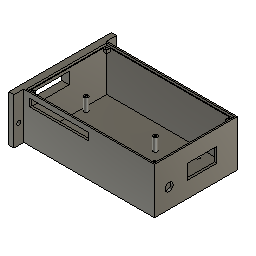
ComputeControlModule v6 (Autodesk Fusion 360 design; units mm, degrees)
Autodesk Fusion 360 part; units mm, degrees
sketch "Sketch1" plane through (0, 0, 0) normal (0, 0, 1) x (1, 0, 0)
  line L0 (0, 0) -> (178, 0)
  line L1 (178, 0) -> (178, 113)
  line L2 (178, 113) -> (0, 113)
  line L3 (0, 113) -> (0, 0)
  dimension "d1" = 178
  dimension "d2" = 113
  constraint horizontal L0
  constraint vertical L1
  constraint horizontal L2
  constraint vertical L3
  constraint coincident L0.start L3.end
  measures "d1" distance of L0.start L0.end
  measures "d2" distance of L0.start L2.end
extrude "Extrude1" add sketch "Sketch1" along normal blind 3
extrude "Extrude2" add 1 faces at (59.3333, 37.6667, 3) along direction (0, 0, 1) blind 60 thin wall 3 inside
sketch "Sketch2" plane through (0, 0, 0) normal (-1, 0, 0) x (0, -1, 0)
  line L0 (-113, 0) -> (0, 0)
  line L1 (0, 0) -> (0, 63)
  line L2 (0, 63) -> (-113, 63)
  line L3 (-113, 63) -> (-113, 0)
  line L4 (13.35, 0) -> (-126.35, 0)
  line L5 (-126.35, 0) -> (-126.35, 63)
  line L6 (-126.35, 63) -> (13.35, 63)
  line L7 (13.35, 63) -> (13.35, 0)
  line L8 (13.35, 0) -> (-126.35, 63) construction
  line L9 (-126.35, 0) -> (13.35, 63) construction
  point P0 (-56.5, 31.5)
  dimension "d8" = 139.7
  dimension "d9" = 63
  constraint horizontal L4
  constraint perpendicular L4 L5
  constraint parallel L4 L6
  constraint parallel L5 L7
  constraint coincident L8 P0
  constraint coincident L9 P0
  measures "d8" distance of L5.end L6.end
  measures "d9" distance of L4.end L5.end
extrude "Extrude3" add sketch "Sketch2" along normal blind 7
sketch "Sketch3" plane through (-7, 0, 0) normal (-1, 0, 0) x (0, -1, 0)
  line L0 (13.35, 63) -> (-126.35, 63)
  line L1 (-126.35, 63) -> (-126.35, 0)
  line L2 (-126.35, 0) -> (13.35, 0)
  line L3 (13.35, 0) -> (13.35, 63)
  point P0 (-120, 26.5)
  point P1 (7, 26.5)
hole "Hole1" at (-7, 120, 26.5) at (-7, -7, 26.5) direction (1, 0, 0) diameter 5.5 depth 12 tip angle 118
sketch "Sketch15" plane through (0, 0, 3) normal (0, 0, 1) x (-1, 0, 0)
  line L0 (-175, -110) -> (-3, -110)
  line L1 (-3, -110) -> (-3, -3)
  line L2 (-3, -3) -> (-175, -3)
  line L3 (-175, -3) -> (-175, -110)
  circle A0 centre (-102, -8) radius 3
  circle A1 centre (-102, -77) radius 3
  circle A2 centre (-8, -8) radius 3
  circle A3 centre (-8, -77) radius 3
  point P0 (-8, -8)
  point P1 (-8, -77)
  point P2 (-102, -8)
  point P3 (-102, -77)
  dimension "d103" = 6
  dimension "d104" = 6
  dimension "d105" = 6
  dimension "d106" = 6
  constraint coincident P2 A0.centre
  constraint coincident P3 A1.centre
  constraint coincident P0 A2.centre
  constraint coincident P1 A3.centre
  measures "d103" diameter of A0
  measures "d104" diameter of A1
  measures "d105" diameter of A2
  measures "d106" diameter of A3
extrude "Extrude13" add sketch "Sketch15" along normal blind 17 contours A0 | A1 | A2 | A3
sketch "Sketch16" plane through (0, 0, 20) normal (0, 0, 1) x (-1, 0, 0)
  circle A0 centre (-102, -8) radius 3
  point P0 (-102, -8)
  point P1 (-8, -8)
  point P2 (-8, -77)
  point P3 (-102, -77)
  constraint coincident P0 A0.centre
hole "Hole14" at (102, 77, 20) at (102, 8, 20) at (8, 8, 20) at (8, 77, 20) direction (0, 0, -1) diameter 2.75 depth 10 tip angle 180
sketch "Sketch17" plane through (0, 0, 3) normal (0, 0, 1) x (-1, 0, 0)
  circle A0 centre (-102, -77) radius 3
  circle A1 centre (-102, -8) radius 3
  circle A2 centre (-8, -77) radius 3
  circle A3 centre (-8, -8) radius 3
  line L0 (-175, -110) -> (-3, -110)
  line L1 (-3, -110) -> (-3, -3)
  line L2 (-3, -3) -> (-175, -3)
  line L3 (-175, -3) -> (-175, -110)
  circle A4 centre (-139, -8) radius 3
  circle A5 centre (-139, -98) radius 3
  point P0 (-139, -8)
  point P1 (-139, -98)
  dimension "d112" = 6
  dimension "d113" = 6
  constraint vertical P0 P1
  constraint coincident P0 A4.centre
  constraint coincident P1 A5.centre
  measures "d112" diameter of A4
  measures "d113" diameter of A5
extrude "Extrude14" add sketch "Sketch17" along normal blind 3 contours A4 | A5
sketch "Sketch18" plane through (0, 0, 6) normal (0, 0, 1) x (-1, 0, 0)
  circle A0 centre (-139, -8) radius 3
  point P0 (-139, -8)
  point P1 (-139, -98)
  constraint coincident P0 A0.centre
  constraint vertical P0 P1
hole "Hole15" at (139, 8, 6) at (139, 98, 6) direction (0, 0, -1) diameter 2.75 depth 4 tip angle 180
sketch "Sketch12" plane through (0, 0, 63) normal (0, 0, 1) x (-1, 0, 0)
  line L0 (-3, -110) -> (-175, -110)
  line L1 (-175, -110) -> (-175, -3)
  line L2 (-175, -3) -> (-3, -3)
  line L3 (-3, -3) -> (-3, -110)
  line L4 (0, 0) -> (-178, 0)
  line L5 (-178, 0) -> (-178, -113)
  line L6 (-178, -113) -> (0, -113)
  line L7 (-2, -111) -> (-176, -111)
  line L8 (-176, -111) -> (-176, -2)
  line L9 (-176, -2) -> (-2, -2)
  line L10 (-2, -2) -> (-2, -111)
  line L11 (0, -113) -> (0, -126.35)
  line L12 (0, -126.35) -> (7, -126.35)
  line L13 (7, -126.35) -> (7, 13.35)
  line L14 (7, 13.35) -> (0, 13.35)
  line L15 (0, 13.35) -> (0, 0)
  constraint horizontal L7
  constraint vertical L8
  constraint horizontal L9
  constraint vertical L10
extrude "Extrude11" cut sketch "Sketch12" against normal blind 3 contours L7 L8 L9 L10
ref_plane "WorkPlane1" through (85.5, 56.5, 61) normal (0, 0, 1) x (1, 0, 0)
sketch "Sketch13" plane through (0, 0, 61) normal (0, 0, 1) x (1, 0, 0)
  line L0 (3, 3) -> (8, 3)
  line L1 (8, 3) -> (8, 8)
  line L2 (8, 8) -> (3, 8)
  line L3 (3, 8) -> (3, 3)
  line L4 (3, 110) -> (8, 110)
  line L5 (8, 110) -> (8, 105)
  line L6 (8, 105) -> (3, 105)
  line L7 (3, 105) -> (3, 110)
  line L8 (175, 3) -> (170, 3)
  line L9 (170, 3) -> (170, 8)
  line L10 (170, 8) -> (175, 8)
  line L11 (175, 8) -> (175, 3)
  line L12 (175, 110) -> (170, 110)
  line L13 (170, 110) -> (170, 105)
  line L14 (170, 105) -> (175, 105)
  line L15 (175, 105) -> (175, 110)
  dimension "d90" = 5
  dimension "d91" = 5
  dimension "d92" = 5
  dimension "d93" = 5
  dimension "d94" = 5
  dimension "d95" = 5
  dimension "d96" = 5
  dimension "d97" = 5
  constraint horizontal L0
  constraint vertical L1
  constraint horizontal L2
  constraint vertical L3
  constraint horizontal L4
  constraint vertical L5
  constraint horizontal L6
  constraint vertical L7
  constraint horizontal L8
  constraint vertical L9
  constraint horizontal L10
  constraint vertical L11
  constraint horizontal L12
  constraint vertical L13
  constraint horizontal L14
  constraint vertical L15
  measures "d90" distance of L0.start L0.end
  measures "d91" distance of L0.start L2.end
  measures "d92" distance of L4.start L4.end
  measures "d93" distance of L4.start L6.end
  measures "d94" distance of L8.start L8.end
  measures "d95" distance of L8.start L10.end
  measures "d96" distance of L12.start L12.end
  measures "d97" distance of L12.start L14.end
extrude "Extrude12" add sketch "Sketch13" against normal blind 5
sketch "Sketch14" plane through (0, 0, 60) normal (0, 0, 1) x (-1, 0, 0)
  line L0 (-3, -8) -> (-3, -105)
  line L1 (-8, -110) -> (-170, -110)
  line L2 (-175, -105) -> (-175, -8)
  line L3 (-170, -3) -> (-8, -3)
  line L4 (-2, -2) -> (-176, -2)
  line L5 (-176, -2) -> (-176, -111)
  line L6 (-176, -111) -> (-2, -111)
  line L7 (-2, -111) -> (-2, -2)
  line L8 (-8, -3) -> (-3, -3)
  line L9 (-3, -3) -> (-3, -8)
  line L10 (-3, -105) -> (-3, -110)
  line L11 (-3, -110) -> (-8, -110)
  line L12 (-170, -110) -> (-175, -110)
  line L13 (-175, -110) -> (-175, -105)
  line L14 (-175, -8) -> (-175, -3)
  line L15 (-175, -3) -> (-170, -3)
  point P0 (-5.5, -5.5)
  point P1 (-5.5, -107.5)
  point P2 (-172.5, -107.5)
  point P3 (-172.5, -5.5)
hole "Hole13" at (172.5, 5.5, 60) at (5.5, 107.5, 60) at (5.5, 5.5, 60) at (172.5, 107.5, 60) direction (0, 0, -1) diameter 2.75 depth 6 tip angle 180
sketch "Sketch19" plane through (178, 0, 0) normal (1, 0, 0) x (0, 1, 0)
  line L0 (0, 0) -> (113, 0)
  line L1 (113, 0) -> (113, 63)
  line L2 (113, 63) -> (0, 63)
  line L3 (0, 63) -> (0, 0)
  point P0 (20, 26.5)
hole "Hole16" at (178, 20, 26.5) direction (-1, 0, 0) diameter 11 depth 10 tip angle 180
sketch "Sketch20" plane through (178, 0, 0) normal (1, 0, 0) x (0, 1, 0)
  circle A0 centre (20, 26.5) radius 5.5
  line L0 (0, 0) -> (113, 0)
  line L1 (113, 0) -> (113, 63)
  line L2 (113, 63) -> (0, 63)
  line L3 (0, 63) -> (0, 0)
  line L4 (45.0125, 22.0134, -3.3761) -> (85.0125, 22.0134, -3.3761)
  line L5 (85.0125, 22.0134, -3.3761) -> (85.0125, 41.9931, -2.4734)
  line L6 (85.0125, 41.9931, -2.4734) -> (45.0125, 41.9931, -2.4734)
  line L7 (45.0125, 41.9931, -2.4734) -> (45.0125, 22.0134, -3.3761)
  line L8 (45.0125, 22.0134, -3.3761) -> (85.0125, 41.9931, -2.4734) construction
  line L9 (85.0125, 22.0134, -3.3761) -> (45.0125, 41.9931, -2.4734) construction
  point P0 (65.0125, 32.0033)
  dimension "d122" = 40
  dimension "d123" = 20
extrude "Extrude15" cut sketch "Sketch20" along normal blind 12 and the other way blind 10 contours L4 L5 L6 L7 in plane through (173.6382, 0, 0.1971) normal (0.998981, 0, -0.045135)
move_face "OffsetFaces1" offset -1 4 faces at (4.6667, 6.3333, 61) (4.6667, 108.3333, 61) (171.6667, 108.3333, 61) (173.3333, 4.6667, 61)
sketch "Sketch22" plane through (3, 0, 0) normal (1, 0, 0) x (0, 1, 0)
  line L0 (8, 56) -> (3, 56)
  line L1 (3, 56) -> (3, 3)
  line L2 (3, 3) -> (110, 3)
  line L3 (110, 3) -> (110, 56)
  line L4 (110, 56) -> (105, 56)
  line L5 (105, 56) -> (105, 60)
  line L6 (105, 60) -> (8, 60)
  line L7 (8, 60) -> (8, 56)
  line L8 (3, 56, 5) -> (59, 56, 5)
  line L9 (59, 56, 5) -> (59, 40, 5)
  line L10 (59, 40, 5) -> (3, 40, 5)
  line L11 (3, 40, 5) -> (3, 56, 5)
  point P0 (3, 56)
  dimension "d127" = 56
  dimension "d128" = 16
  constraint coincident P0 L0.end
extrude "Extrude16" cut sketch "Sketch22" against normal blind 15 contours L8 L9 L10 L11 in plane through (8, 0, 0) normal (1, 0, 0)
sketch "Sketch23" plane through (0, 3, 0) normal (0, 1, 0) x (-1, 0, 0)
  line L0 (7, 56) -> (-8, 56)
  line L1 (-8, 56) -> (-8, 60)
  line L2 (-8, 60) -> (-170, 60)
  line L3 (-170, 60) -> (-170, 56)
  line L4 (-170, 56) -> (-175, 56)
  line L5 (-175, 56) -> (-175, 3)
  line L6 (-175, 3) -> (-3, 3)
  line L7 (-3, 3) -> (-3, 40)
  line L8 (-3, 40) -> (7, 40)
  line L9 (7, 40) -> (7, 56)
  line L10 (-8, 56) -> (-88, 56)
  line L11 (-88, 56) -> (-88, 46)
  line L12 (-88, 46) -> (-8, 46)
  line L13 (-8, 46) -> (-8, 56)
  dimension "d131" = 80
  dimension "d132" = 10
  constraint horizontal L10
  constraint vertical L11
  constraint horizontal L12
  constraint vertical L13
  constraint coincident L0.end L1.start
  measures "d131" distance of L0.end L10.end
  measures "d132" distance of L0.end L12.end
extrude "Extrude17" cut sketch "Sketch23" against normal blind 10 contours L10 L11 L12 L13
